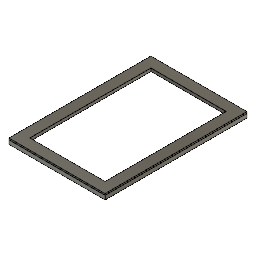
photo_frame10x15 (Autodesk Fusion 360 design; units mm, degrees)
Autodesk Fusion 360 part; units mm, degrees
sketch "Sketch1" plane through (0, 0, 0) normal (0, 0, 1) x (1, 0, 0)
  line L0 (-55, 60) -> (47, 60)
  line L1 (47, 60) -> (47, -92)
  line L2 (47, -92) -> (-55, -92)
  line L3 (-55, -92) -> (-55, 60)
  line L4 (-50, 55) -> (42, 55)
  line L5 (42, 55) -> (42, -87)
  line L6 (42, -87) -> (-50, -87)
  line L7 (-50, -87) -> (-50, 55)
  line L8 (-56.6, 61.6) -> (48.6, 61.6)
  line L9 (48.6, 61.6) -> (48.6, -93.6)
  line L10 (48.6, -93.6) -> (-56.6, -93.6)
  line L11 (-56.6, -93.6) -> (-56.6, 61.6)
  dimension "d1" = 102
  dimension "d2" = 152
  dimension "d3" = 105.2
  dimension "d4" = 155.2
  dimension "d5" = 1.6
  dimension "d6" = 1.6
  constraint horizontal L0
  constraint vertical L1
  constraint horizontal L2
  constraint vertical L3
  constraint horizontal L4
  constraint vertical L5
  constraint horizontal L6
  constraint vertical L7
  constraint horizontal L8
  constraint vertical L9
  constraint horizontal L10
  constraint vertical L11
  measures "d1" distance of L0.start L0.end
  measures "d2" distance of L0.start L2.end
  measures "d3" distance of L8.start L8.end
  measures "d4" distance of L8.start L10.end
  measures "d5" distance of L3 L11
  measures "d6" distance of L0 L8
extrude "Extrude1" add sketch "Sketch1" against normal blind 1.6 contours L0 L1 L2 L3 | L8 L9 L10 L11 makes body 1 in component "Component"
extrude "Extrude2" add sketch "Sketch1" along normal blind 3 contours L8 L9 L10 L11 bodies 1 in component "Component"
sketch "Sketch2" plane through (0, 0, 0) normal (0, 0, 1) x (1, 0, 0)
  line L0 (-55, 60) -> (46.8, 60)
  line L1 (46.8, 60) -> (46.8, -91.8)
  line L2 (46.8, -91.8) -> (-55, -91.8)
  line L3 (-55, -91.8) -> (-55, 60)
  line L4 (-45, 50) -> (37, 50)
  line L5 (37, 50) -> (37, -82)
  line L6 (37, -82) -> (-45, -82)
  line L7 (-45, -82) -> (-45, 50)
  dimension "d11" = 101.8
  dimension "d12" = 151.8
  dimension "d13" = 82
  dimension "d14" = 132
  constraint horizontal L0
  constraint vertical L1
  constraint horizontal L2
  constraint vertical L3
  constraint horizontal L4
  constraint vertical L5
  constraint horizontal L6
  constraint vertical L7
  measures "d11" distance of L0.start L0.end
  measures "d12" distance of L0.start L2.end
  measures "d13" distance of L4.start L4.end
  measures "d14" distance of L4.start L6.end
extrude "Extrude1'" add sketch "Sketch2" along normal blind 1.6 separate body makes body 2 in component "Component'"
move_face "MoveFace1" by (0, 0, 1.4) 1 faces at (-51.6667, 6.0667, 1.6) on bodies 2 in component "Component'"
fillet "Fillet1" radius 2 4 edges at (-55, 60, 1.5) (46.8, 60, 1.5) (46.8, -91.8, 1.5) (-55, -91.8, 1.5) on bodies 2 in component "Component'"
sketch "Sketch1 (2)" plane through (0, 0, 3) normal (0, 0, 1) x (-1, 0, 0) in component "Component'"
  arc A0 (55, 89.8) -> (53, 91.8) centre (53, 89.8) ccw
  line L0 (53, 91.8) -> (-44.8, 91.8)
  arc A1 (-44.8, 91.8) -> (-46.8, 89.8) centre (-44.8, 89.8) ccw
  line L1 (-46.8, 89.8) -> (-46.8, -58)
  arc A2 (-46.8, -58) -> (-44.8, -60) centre (-44.8, -58) ccw
  line L2 (-44.8, -60) -> (53, -60)
  arc A3 (53, -60) -> (55, -58) centre (53, -58) ccw
  line L3 (55, -58) -> (55, 89.8)
  line L4 (-37, 82) -> (45, 82)
  line L5 (45, 82) -> (45, -50)
  line L6 (45, -50) -> (-37, -50)
  line L7 (-37, -50) -> (-37, 82)
  line L8 (56.5668, -61.4819) -> (-48.6332, -61.4819)
  line L9 (-48.6332, -61.4819) -> (-48.6332, 93.7181)
  line L10 (-48.6332, 93.7181) -> (56.5668, 93.7181)
  line L11 (56.5668, 93.7181) -> (56.5668, -61.4819)
  dimension "d19" = 105.2
  dimension "d20" = 155.2
  constraint horizontal L8
  constraint vertical L9
  constraint horizontal L10
  constraint vertical L11
  measures "d19" distance of L8.start L8.end
  measures "d20" distance of L8.start L10.end
extrude "Extrude2'" add sketch "Sketch1 (2)" along normal blind 1.6 contours A0 L0 A1 L1 A2 L2 A3 L3 | L8 L9 L10 L11 bodies 2 in component "Component'"
move_face "MoveFace2" by (0, 0, 1.2) 1 faces at (-51.6667, 6.0667, 0) on bodies 2 in component "Component'"
component "Component" placed x (1, 0, 0) y (0, 1, 0) z (0, 0, 1) at (0, 0, 0)
component "Component'" placed x (1, 0, 0) y (0, 1, 0) z (0, 0, 1) at (0, 0, 0)
